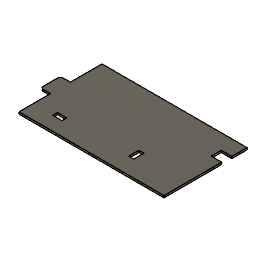
Control board - middle high plate v2 (Autodesk Fusion 360 design; units mm, degrees)
Autodesk Fusion 360 part; units mm, degrees
sketch "Sketch1" plane through (0, 0, 0) normal (0, 0, 1) x (1, 0, 0)
  line L0 (-0.9, 44.4476) -> (72, 44.4476)
  line L1 (72, 44.4476) -> (72, 2.6476)
  line L2 (72, 2.6476) -> (-0.9, 2.6476)
  line L3 (-0.9, 2.6476) -> (-0.9, 44.4476)
  line L4 (-0.9, 23.5476) -> (72, 23.5476) construction
  line L5 (-0.9, 28.5476) -> (-4.6, 28.5476)
  line L6 (-5.9, 27.2476) -> (-5.9, 19.8476)
  line L7 (-4.6, 18.5476) -> (-0.9, 18.5476)
  line L8 (-0.9, 18.5476) -> (-0.9, 28.5476)
  arc A0 (-4.6, 28.5476) -> (-5.9, 27.2476) centre (-4.6, 27.2476) ccw
  arc A1 (-5.9, 19.8476) -> (-4.6, 18.5476) centre (-4.6, 19.8476) ccw
  line L9 (72, 36.7476) -> (66.7, 36.7476)
  line L10 (66.7, 36.7476) -> (66.7, 31.7476)
  line L11 (66.7, 31.7476) -> (72, 31.7476)
  line L12 (72, 31.7476) -> (72, 36.7476)
  line L13 (46, 16.0476) -> (48.5, 16.0476)
  line L14 (48.5, 16.0476) -> (48.5, 11.0476)
  line L15 (48.5, 11.0476) -> (46, 11.0476)
  line L16 (46, 11.0476) -> (46, 16.0476)
  line L17 (9.1, 12.0476) -> (13.7, 12.0476)
  line L18 (13.7, 12.0476) -> (13.7, 9.7476)
  line L19 (13.7, 9.7476) -> (9.1, 9.7476)
  line L20 (9.1, 9.7476) -> (9.1, 12.0476)
  point P0 (-5.9, 28.5476)
  point P1 (-5.9, 18.5476)
  dimension "d1" = 72.9
  dimension "d2" = 41.8
  dimension "d7" = 10
  dimension "d8" = 5
  dimension "d9" = 1.3
  dimension "d10" = 5.3
  dimension "d11" = 5
  dimension "d12" = 7.7
  dimension "d13" = 2.5
  dimension "d14" = 5
  dimension "d15" = 8.4
  dimension "d16" = 23.5
  dimension "d17" = 2.3
  dimension "d18" = 7.1
  dimension "d19" = 10
  dimension "d20" = 14.6
  constraint horizontal L0
  constraint vertical L1
  constraint horizontal L2
  constraint vertical L3
  constraint midpoint L3 L4.start
  constraint midpoint L1 L4.end
  constraint horizontal L5
  constraint vertical L6
  constraint horizontal L7
  constraint vertical L8
  constraint coincident L3 L5.start
  constraint symmetric L4 L5 L7
  constraint coincident P0 L5
  constraint coincident P0 L6
  constraint tangent L5 A0
  constraint tangent L6 A0
  constraint coincident P1 L6
  constraint coincident P1 L7
  constraint tangent L6 A1
  constraint tangent L7 A1
  constraint equal A0 A1
  constraint horizontal L9
  constraint vertical L10
  constraint horizontal L11
  constraint vertical L12
  constraint coincident L1 L9.start
  constraint horizontal L13
  constraint vertical L14
  constraint horizontal L15
  constraint vertical L16
  constraint horizontal L17
  constraint vertical L18
  constraint horizontal L19
  constraint vertical L20
  measures "d1" distance of L0.start L0.end
  measures "d2" distance of L0.end L1.end
  measures "d7" distance of P0 P1
  measures "d8" distance of L5.start P0
  measures "d9" radius of A0
  measures "d10" distance of L9.start L9.end
  measures "d11" distance of L9.end L10.end
  measures "d12" distance of L0 L9
  measures "d13" distance of L13.start L13.end
  measures "d14" distance of L13.end L14.end
  measures "d15" distance of L2 L15
  measures "d16" distance of L1 L14
  measures "d17" distance of L17.start L19.end
  measures "d18" distance of L2 L19
  measures "d19" distance of L3 L20
  measures "d20" distance of L3 L18
extrude "Extrude1" add sketch "Sketch1" along normal blind 1 contours L0 L1 L2 L3 L8 L9 L10 L11 | L3 L5 L6 L7 L8 A0 A1
